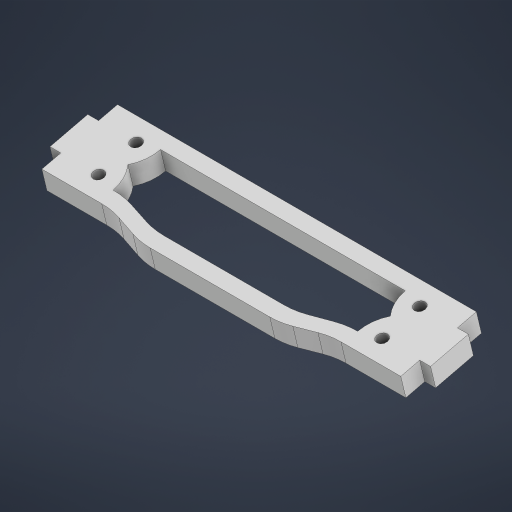
# Autodesk Inventor part: motor_mount
Saved by Autodesk Inventor 2024 (Build 280153000, 153)
## iProperties
Created: 2022-03-25
Part Number: motor_mount
Material: Generic
Document SubType Name: Modeling
Designer: kardo
Density: 1 g/cm^3
Appearance: Default
Mass: 7.4065 g
Surface Area: 52.0175 cm^2
Volume: 7.4065 cm^3
Author: kardo
Autodesk Inventor part; units mm, degrees
ref_plane "YZ Plane" through (0, 0, 0) normal (1, 0, 0) x (0, 1, 0)
ref_plane "XZ Plane" through (0, 0, 0) normal (0, 1, 0) x (-1, 0, 0)
ref_plane "XY Plane" through (0, 0, 0) normal (0, 0, 1) x (1, 0, 0)
derived "parameters_frame.ipt"
derived "stencil_frame.ipt"
sketch "sk_cowl_joint_locations" plane through (54.6, 0, 0) normal (1, 0, 0) x (0, 1, 0)
  line L0 (-345, 16.32) -> (-262.2001, 18.586) construction
  arc A0 (-262.2001, 18.586) -> (-241.5001, 19.2432) centre (-326.8578, 2381.2399) ccw construction
  line L1 (-241.5001, 19.2432) -> (11.22, 28.376) construction
  arc A1 (36.465, 28.832) -> (11.22, 28.376) centre (36.465, -670.197) ccw construction
  line L2 (36.465, 28.832) -> (112.2, 28.832) construction
  line L3 (94.8, 29.632) -> (36.465, 29.632) construction
  arc A2 (36.465, 29.632) -> (11.1911, 29.1755) centre (36.465, -670.197) ccw construction
  line L4 (11.1911, 29.1755) -> (-241.529, 20.0427) construction
  arc A3 (-262.222, 19.3857) -> (-241.529, 20.0427) centre (-326.8578, 2381.2399) ccw construction
  line L5 (-262.222, 19.3857) -> (-345, 17.1203) construction
  line L6 (-230.0001, 3089.1136) -> (-230.0001, -1866.0023) construction
  line L7 (-114.9999, 3089.1136) -> (-114.9999, -1866.0023) construction
  line L8 (-345, 3089.1136) -> (-345, -1866.0023) construction
  line L9 (0, 3089.1136) -> (0, -1866.0023) construction
  line L10 (-230.0001, 44.8681) -> (-230.0001, 20.4593) construction
  line L11 (-114.9999, 49.7658) -> (-114.9999, 24.6152) construction
  line L12 (-345, 17.1203) -> (-345, 17.1203)
  line L13 (-345, 17.1203) -> (-345, 36.7228) construction
  line L14 (-850.7464, 3011.9134) -> (325.2296, -1886.3794) construction
  line L15 (-344.7454, 36.7228) -> (-345, 39.712) construction
  line L16 (0, 51.4) -> (0, 28.7711) construction
  line L17 (-144.5331, 44.6212) -> (-139.5174, 23.7292) construction
  line L18 (-134.9371, 30.3529) -> (-140.7713, 28.9522) construction
  line L19 (-137.4449, 40.7989) -> (-143.2792, 39.3982) construction
  spline S0 degree 2 poles (-345, 39.712) (-172.656, 54.3934) (0, 54.4) knots 0 0 0 1 1 1
  spline S1 degree 3 poles (0, 54.4) (37.026, 54.4) (80.784, 47.9917) (112.2, 37.536) knots 1 1 1 1 2 2 2 2
  spline S2 degree 3 poles (111.2526, 34.6895) (106.0906, 36.4075) (96.4401, 39.2282) (84.5011, 42.0313) (75.2591, 43.9395) (68.9709, 45.1125) (60.9945, 46.449) (54.5373, 47.4124) (46.413, 48.4791) (39.8882, 49.2203) (31.7426, 50.0013) (25.2514, 50.5076) (17.2112, 50.9875) (9.2661, 51.3118) (3.0567, 51.4) (0, 51.4) knots 1 1 1 1 1.166667 1.291667 1.333333 1.416667 1.458333 1.541667 1.583333 1.666667 1.708333 1.791667 1.833333 1.916667 2 2 2 2
  spline S3 degree 3 poles (0, 51.4) (-19.1698, 51.3993) (-52.712, 51.1604) (-91.0357, 50.4121) (-119.7742, 49.6473) (-138.931, 49.0355) (-162.8744, 48.1436) (-182.0269, 47.3282) (-205.9648, 46.1816) (-225.113, 45.1626) (-249.0455, 43.7615) (-268.1894, 42.5387) (-292.1166, 40.883) (-316.041, 39.1) (-335.1777, 37.5379) (-344.7454, 36.7228) knots 0 0 0 0 0.166667 0.291667 0.333333 0.416667 0.458333 0.541666 0.583333 0.666666 0.708333 0.791666 0.833333 0.916666 1 1 1 1
  line L20 (-144.5331, 44.6212) -> (-138.6989, 46.0219) construction
  line L21 (-139.5174, 23.7292) -> (-133.6831, 25.1299) construction
  line L22 (-138.6989, 46.0219) -> (-138.9044, 52.0184) construction
  point P0 (0, 0)
  point P1 (-345, 26.9216)
  point P2 (-230.0001, 32.6637)
  point P3 (-114.9999, 37.1905)
  point P4 (0, 40.0855)
  point P5 (0, 40.0855)
ref_plane "plane_motor_mount" through (0, -127.65, 0) normal (0, 0.9723699, 0.2334454) x (-1, 0, 0)
ref_plane "plane_cowl_right" through (54.6, 0, 0) normal (1, 0, 0) x (0, 1, 0)
ref_plane "plane_symmetry" through (0, 0, 0) normal (1, 0, 0) x (0, 1, 0)
sketch "sk_drivetrain_profile" plane through (6, 0, 0) normal (1, 0, 0) x (0, 1, 0)
  line L0 (-529.1844, 0) -> (410.1064, 0) construction
  line L1 (-345, 3089.1136) -> (-345, -1866.0023) construction
  line L2 (0, 3089.1136) -> (0, -1866.0023) construction
  line L3 (-140.3859, 53.0487) -> (-133.8494, 25.8223)
  line L4 (-377, 0) -> (-313.1973, 5.0214)
  line L5 (-137.1176, 39.4355) -> (-233.3061, 16.3427)
  line L6 (-296.4782, 6.3372) -> (-264.4984, 8.8541) construction
  line L7 (-264.4984, 8.8541) -> (-233.3061, 16.3427) construction
  line L8 (-133.8494, 25.8223) -> (-133.8494, 20.8223) construction
  line L9 (-313.1973, 5.0214) -> (-296.4782, 6.3372)
  line L10 (-850.7464, 3011.9134) -> (325.2296, -1886.3794) construction
  line L11 (-233.9547, 19.044) -> (-137.7662, 42.1369) construction
  line L12 (-136.4691, 36.7341) -> (-232.6576, 13.6413) construction
  line L13 (-233.9547, 19.044) -> (-232.6576, 13.6413) construction
  line L14 (0, 21.3303) -> (-241.5001, 18.9703) construction
  line L15 (-55.7851, 21.5852) -> (-309.9218, 19.1017) construction
  spline S0 degree 2 poles (-296.4782, 6.3372) (-264.4984, 8.8541) (-233.3061, 16.3427) knots 1 1 1 2 2 2
  point P0 (0, 0)
  point P1 (-221.5492, 19.1653)
  point P2 (-209.1437, 19.2865)
  point P3 (-205.6699, 20.1205)
sketch "sk_base" plane through (0, -127.65, 0) normal (0, 0.9723699, 0.2334454) x (-1, 0, 0)
  line L0 (-54.6, -1324.4284) -> (-54.6, 2990.003) construction
  line L1 (0, -1324.4284) -> (0, 2990.003) projected
  line L2 (0, 50.5561) -> (-16.5333, 50.5561)
  line L3 (-49.6, 47.3296) -> (-49.6, 41.9582)
  line L4 (-49.6, 41.9582) -> (-52.6, 41.9582)
  line L5 (-52.6, 41.9582) -> (-52.6, 31.2153)
  line L6 (-52.6, 31.2153) -> (-49.6, 31.2153)
  line L7 (-49.6, 31.2153) -> (-49.6, 25.8439)
  line L8 (-49.6, 25.8439) -> (0, 25.8439)
  line L9 (-33.0667, 47.3296) -> (-49.6, 47.3296)
  arc A0 (-33.0667, 47.3296) -> (-27.4972, 48.1405) centre (-33.0667, 66.8625) ccw
  arc A1 (-16.5333, 50.5561) -> (-22.1028, 49.7452) centre (-16.5333, 31.0232) ccw
  line L10 (-27.4972, 48.1405) -> (-22.1028, 49.7452)
  line L11 (-33.0667, 47.3296) -> (-27.4972, 48.1405) construction
  line L12 (-22.1028, 49.7452) -> (-16.5333, 50.5561) construction
  line L13 (-33.0667, 47.3296) -> (-16.5333, 47.3296) construction
  line L14 (-16.5333, 47.3296) -> (-16.5333, 50.5561) construction
  point P0 (0, -29.7993)
  point P1 (-54.6, 41.9582)
  point P2 (-54.6, 31.2153)
  point P3 (-54.6, 47.3296)
  point P4 (-54.6, 25.8439)
  point P5 (-6, 40.5561)
  dimension "d2" = 5
  dimension "d3" = 3
  dimension "d26" = 10
  constraints: 26 end point, 7 perpendicular, 6 point on line, 4 equal length, 4 point on circle, 4 tangent, 2 centre point, 2 parallel, 1 collinear
  measures "d2" distance between parallel lines of L0 L3
  measures "d3" distance between parallel lines of L3 L5
  measures "d26" distance from line of point (-6, 40.556) L2
extrude "thicken" add sketch "sk_base" against normal blind 6
sketch "sk_cut" plane through (0, -127.65, 0) normal (0, 0.9723699, 0.2334454) x (-1, 0, 0)
  line L0 (-49.6, 25.8439) -> (0, 25.8439) construction
  line L1 (0, 25.8439) -> (0, 50.5561) projected
  line L2 (0, 50.5561) -> (-16.5333, 50.5561) construction
  line L3 (-49.6, 47.3296) -> (-49.6, 41.9582) construction
  line L4 (-49.6, 41.9582) -> (-52.6, 41.9582) construction
  line L5 (-52.6, 41.9582) -> (-52.6, 31.2153) construction
  line L6 (-52.6, 31.2153) -> (-49.6, 31.2153) construction
  line L7 (-49.6, 31.2153) -> (-49.6, 25.8439) construction
  line L8 (0, 25.8439) -> (0, 50.5561) projected
  line L9 (0, 29.8439) -> (-33.8, 29.8439)
  arc A0 (-33.8, 29.8439) -> (-36.2542, 36.5868) centre (-44.29, 29.8439) ccw
  arc A1 (-36.2542, 36.5868) -> (-33.8, 43.3296) centre (-44.29, 43.3296) ccw
  circle A2 centre (-39.2, 41.9296) radius 1.5
  circle A3 centre (-39.2, 31.2439) radius 1.5
  line L10 (-44.6, 47.3296) -> (-44.6, 25.8439) construction
  line L11 (-33.8, 43.3296) -> (-33.8, 29.8439) construction
  line L12 (-39.2, 31.2439) -> (-44.6, 31.2439) construction
  line L13 (-39.2, 31.2439) -> (-39.2, 25.8439) construction
  line L14 (-39.2, 41.9296) -> (-39.2, 47.3296) construction
  line L15 (-39.2, 41.9296) -> (-44.6, 41.9296) construction
  arc A4 (-16.5333, 50.5561) -> (-22.1028, 49.7452) centre (-16.5333, 31.0232) ccw construction
  line L16 (-22.1028, 49.7452) -> (-27.4972, 48.1405) construction
  arc A5 (-33.0667, 47.3296) -> (-27.4972, 48.1405) centre (-33.0667, 66.8625) ccw construction
  line L17 (-33.0667, 47.3296) -> (-49.6, 47.3296) construction
  line L18 (-33.0667, 47.3296) -> (-49.6, 47.3296) construction
  line L19 (0, 50.5561) -> (-16.5333, 50.5561) construction
  line L20 (0, 46.5561) -> (-16.5333, 46.5561)
  line L21 (-16.5333, 50.5561) -> (-16.5333, 46.5561) construction
  arc A6 (-16.5333, 46.5561) -> (-22.3448, 45.7456) centre (-16.5333, 25.316) ccw
  arc A7 (-33.8, 43.3296) -> (-27.9886, 44.1401) centre (-33.8, 64.5697) ccw
  line L22 (-27.9886, 44.1401) -> (-22.3448, 45.7456)
  line L23 (-33.8, 43.3296) -> (-27.9886, 44.1401) construction
  line L24 (-22.3448, 45.7456) -> (-16.5333, 46.5561) construction
  point P0 (0, -29.7993)
  point P1 (-34.4326, 33.4317)
  point P2 (0, 46.5561)
  dimension "d7" = 3
  dimension "d12" = 4
  dimension "d13" = 140
  dimension "d22" = 5
  dimension "d23" = 5.4
  dimension "d24" = 5.4
  dimension "d27" = 4
  dimension "d28" = 4
  constraints: 24 end point, 9 point on circle, 9 point on line, 6 centre point, 4 equal length, 4 perpendicular, 4 tangent, 3 parallel, 2 equal radius, 2 line through centre
  measures "d7" diameter of A2
  measures "d12" distance between parallel lines of L0 L9
  measures "d22" distance between parallel lines of L10 L3
  measures "d23" distance between parallel lines of L10 L13
  measures "d24" distance between parallel lines of L13 L11
  measures "d27" distance from line of L17 L11.start
  measures "d28" distance between parallel lines of L20 L2
extrude "cut" cut sketch "sk_cut" along normal through all both and the other way through all
mirror "mirror" about plane through (0, 0, 0) normal (1, 0, 0)
equation "\"d2\" = cowl_liner_width"
equation "\"d3\" = bulkhead_thickness"
equation "\"d4\" = 2 * bulkhead_thickness"
equation "\"d7\" = drill_motor_mount_diam"
equation "\"d12\" = bulkhead_inset"
equation "\"d22\" = cowl_sealing_width"
equation "\"d23\" = 1.8 * drill_motor_mount_diam"
equation "\"d24\" = 1.8 * drill_motor_mount_diam"
equation "\"d27\" = bulkhead_inset"
equation "\"d28\" = bulkhead_inset"
equation "\"cowl_liner_width\" = 5"
equation "\"bulkhead_thickness\" = 3"
equation "\"drill_motor_mount_diam\" = 3"
equation "\"bulkhead_inset\" = 4"
equation "\"cowl_sealing_width\" = 5"
body "Solid1"
